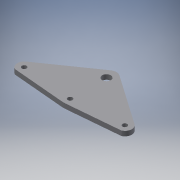
# Autodesk Inventor part: Corpo_Suporte_3_Cabos_Modelo2
Saved by Autodesk Inventor 2018 (Build 220112000, 112)
## iProperties
Created: 2021-08-02
Part Number: Corpo_Suporte_3_Cabos_Modelo2
Material: Generic
Document SubType Name: Modeling
Designer: L08619
Density: 1 g/cm^3
Appearance: Default
Author: L08619
Autodesk Inventor part; units mm, degrees
ref_plane "YZ Plane" through (0, 0, 0) normal (1, 0, 0) x (0, 1, 0)
ref_plane "XZ Plane" through (0, 0, 0) normal (0, 1, 0) x (-1, 0, 0)
ref_plane "XY Plane" through (0, 0, 0) normal (0, 0, 1) x (1, 0, 0)
sketch "Sketch1" plane through (0, 0, 0) normal (0, 0, 1) x (1, 0, 0)
  circle A0 centre (0, 0) radius 20
  circle A1 centre (-235.1359, -149.373) radius 11
  arc A2 (-253.6972, -122.8337) -> (-248.839, -178.7173) centre (-235.1359, -149.373) ccw
  line L0 (-253.6972, -122.8337) -> (-20, 40)
  line L1 (-20, 40) -> (-10, 46.2314) construction
  spline S0 degree 2 poles (-20, 40) (-10, 46.2314) (-0.0129, 46.2314) knots 1 1 1 1.5 1.5 1.5
  line L2 (-0.0129, 87.1559) -> (-0.0129, -290.9336) construction
  line L3 (-10, 46.2314) -> (-0.0129, 46.2314) construction
  circle A3 centre (235.1101, -149.373) radius 11
  arc A4 (248.8132, -178.7173) -> (253.6714, -122.8337) centre (235.1101, -149.373) ccw
  line L4 (253.6714, -122.8337) -> (19.9742, 40)
  line L5 (19.9742, 40) -> (9.9742, 46.2314) construction
  spline S1 degree 2 poles (19.9742, 40) (9.9742, 46.2314) (-0.0129, 46.2314) knots 1 1 1 1.5 1.5 1.5
  line L6 (9.9742, 46.2314) -> (-0.0129, 46.2314) construction
  circle A5 centre (-0.0129, -170) radius 11
  line L7 (248.8132, -178.7173) -> (9.0519, -200)
  arc A6 (-9.0777, -200) -> (9.0519, -200) centre (-0.0129, -97.8799) ccw
  line L8 (-9.0777, -200) -> (-248.839, -178.7173)
  line L9 (-9.0777, -200) -> (9.0519, -200) construction
  dimension "d0" = 40
  dimension "d3" = 22
  dimension "d9" = 40
  dimension "d12" = 120
  dimension "d18" = 22
  dimension "d19" = 170
  dimension "d22" = 30
  constraints: 12 end point, 7 centre point, 6 point on circle, 6 symmetric about line, 3 coincident, 2 point on line, 2 tangent, 1 horizontal, 1 vertical, 8 other
  measures "d0" diameter of A0
  measures "d3" diameter of A1
  measures "d9" vertical distance of L0.end point (0, 0)
  measures "d18" diameter of A5
  measures "d19" distance of point (0, 0) A5.centre
  measures "d22" distance from line of A5.centre L9
extrude "Extrusion2" add sketch "Sketch1" along normal mid plane 22.22
equation "\"d18\" = d3"
body "Solid2"
